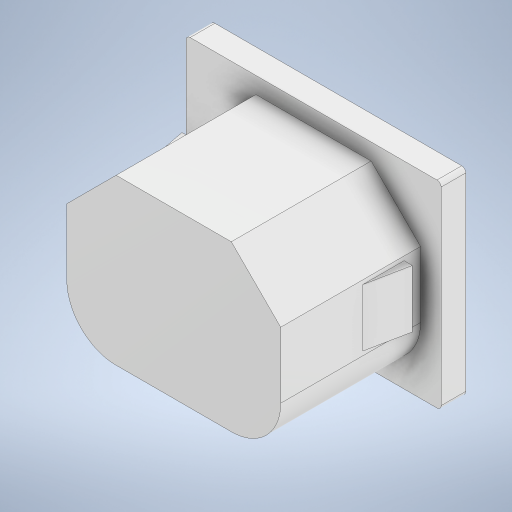
# Autodesk Inventor part: power_socket_24V_2
Saved by Autodesk Inventor 2023 (Build 270158000, 158)
## iProperties
Created: 2023-06-03
Part Number: power_socket_24V_2
Material: ABS Plastic
Document SubType Name: Modeling
Designer: 310611102
Density: 1.06 g/cm^3
Appearance: Smooth - White
Mass: 3.9038 g
Surface Area: 48.2017 cm^2
Volume: 3.68283 cm^3
Author: 310611102
Autodesk Inventor part; units mm, degrees
ref_plane "YZ Plane" through (0, 0, 0) normal (1, 0, 0) x (0, 1, 0)
ref_plane "XZ Plane" through (0, 0, 0) normal (0, 1, 0) x (-1, 0, 0)
ref_plane "XY Plane" through (0, 0, 0) normal (0, 0, 1) x (1, 0, 0)
sketch "Sketch1" plane through (0, 0, 0) normal (0, 0, 1) x (1, 0, 0)
  line L0 (-15.5, 12) -> (15.5, 12)
  line L1 (15.5, 12) -> (15.5, -12)
  line L2 (15.5, -12) -> (-15.5, -12)
  line L3 (-15.5, -12) -> (-15.5, 12)
  line L4 (-15.5, 12) -> (15.5, -12) construction
  line L5 (15.5, 12) -> (-15.5, -12) construction
  point P0 (0, 0)
  dimension "d0" = 24
  dimension "d1" = 31
  constraints: 12 end point, 8 point on line, 2 midpoint, 2 parallel, 1 horizontal, 1 perpendicular
  measures "d0" distance of L5.start L4.end
  measures "d1" distance of L4.start L5.start
extrude "Extrusion1" add sketch "Sketch1" along normal blind 3
fillet "Fillet1" radius 0.5 4 edges at (15.5, 12, 1.5) (15.5, -12, 1.5) (-15.5, -12, 1.5) (-15.5, 12, 1.5)
sketch "Sketch4" plane through (0, 0, 3) normal (0, 0, 1) x (1, 0, 0)
  line L0 (-7, -10) -> (7, -10)
  line L1 (13, -4) -> (13, 4)
  line L2 (7, 10) -> (-7, 10)
  line L3 (-13, 4) -> (-13, -4)
  line L4 (-13, -10) -> (13, 10) construction
  line L5 (13, -10) -> (-13, 10) construction
  arc A0 (-13, -4) -> (-7, -10) centre (-7, -4) ccw
  arc A1 (7, -10) -> (13, -4) centre (7, -4) ccw
  line L6 (-7, 10) -> (-13, 4)
  line L7 (13, 4) -> (7, 10)
  point P0 (0, 0)
  point P1 (0, 0)
  dimension "d13" = 20
  dimension "d14" = 26
  dimension "d41" = 6
  dimension "d42" = 6
  dimension "d43" = 6
  dimension "d44" = 6
  dimension "d45" = 6
  constraints: 16 end point, 16 point on line, 4 point on circle, 4 tangent, 2 centre point, 2 midpoint, 2 parallel, 1 coincident, 1 equal radius, 1 horizontal, 1 perpendicular
  measures "d13" distance of L5.start L4.end
  measures "d14" distance of L4.end L5.end
  measures "d41" radius of A0
  measures "d42" distance of L2.end point (-13, 10)
  measures "d43" distance of L3.start point (-13, 10)
  measures "d44" distance of L1.end point (13, 10)
  measures "d45" distance of L2.start point (13, 10)
extrude "Extrusion4" add sketch "Sketch4" along normal blind 17
sketch "Sketch8" plane through (0, 0, 0) normal (0, 1, 0) x (-1, 0, 0)
  line L0 (-13, 10) -> (-14, 5)
  line L1 (-14, 5) -> (-13, 5)
  line L2 (-15, 3) -> (15, 3) projected
  line L3 (-13, 5) -> (-13, 10)
  line L4 (-13, 3) -> (-13, 20) projected
  point P0 (0, 0)
  dimension "d36" = 2
  dimension "d37" = 1
  dimension "d38" = 5
  constraints: 6 end point, 1 horizontal, 1 point on line, 1 vertical
  measures "d36" distance between parallel lines of L2 L1
  measures "d37" distance of L0.end L1.end
  measures "d38" distance of L1.end L0.start
extrude "Extrusion7" add sketch "Sketch8" along normal mid plane 7
mirror "Mirror1" about plane through (0, 0, 0) normal (1, 0, 0) of "Extrusion7"
sketch "Sketch5" plane through (0, 0, 0) normal (0, 0, -1) x (-1, 0, 0)
  line L0 (-7.5, 8.5) -> (7.5, 8.5)
  line L1 (12.5, 3.5) -> (12.5, -4.5)
  line L2 (8.5, -8.5) -> (-8.5, -8.5)
  line L3 (-12.5, -4.5) -> (-12.5, 3.5)
  line L4 (-12.5, 8.5) -> (12.5, -8.5) construction
  line L5 (12.5, 8.5) -> (-12.5, -8.5) construction
  line L6 (-12.5, 3.5) -> (-7.5, 8.5)
  line L7 (7.5, 8.5) -> (12.5, 3.5)
  arc A0 (-12.5, -4.5) -> (-8.5, -8.5) centre (-8.5, -4.5) ccw
  arc A1 (8.5, -8.5) -> (12.5, -4.5) centre (8.5, -4.5) ccw
  point P0 (0, 0)
  dimension "d18" = 17
  dimension "d19" = 25
  dimension "d20" = 5
  dimension "d21" = 5
  dimension "d22" = 5
  dimension "d23" = 5
  dimension "d24" = 4
  constraints: 16 end point, 8 point on line, 4 point on circle, 4 tangent, 2 centre point, 2 midpoint, 2 parallel, 1 equal radius, 1 horizontal, 1 perpendicular
  measures "d18" distance of L5.start L4.end
  measures "d19" distance of L4.start L5.start
  measures "d20" distance of L3.end L4.start
  measures "d21" distance of L0.start L4.start
  measures "d22" distance of L0.end L5.start
  measures "d23" distance of L1.start L5.start
  measures "d24" radius of A0
extrude "Extrusion5" cut sketch "Sketch5" against normal blind 17
sketch "Sketch7" plane through (0, 0, 17) normal (0, 0, -1) x (-1, 0, 0)
  line L0 (0.5, 3.7551) -> (-0.5, 3.7551)
  line L1 (-0.5, 3.7551) -> (-0.5, 0.5551)
  line L2 (-0.5, 0.5551) -> (0.5, 0.5551)
  line L3 (0.5, 0.5551) -> (0.5, 3.7551)
  line L4 (0.5, 3.7551) -> (-0.5, 0.5551) construction
  line L5 (-0.5, 3.7551) -> (0.5, 0.5551) construction
  line L6 (7.6155, -0.4449) -> (6.6155, -0.4449)
  line L7 (6.6155, -0.4449) -> (6.6155, -3.6449)
  line L8 (6.6155, -3.6449) -> (7.6155, -3.6449)
  line L9 (7.6155, -3.6449) -> (7.6155, -0.4449)
  line L10 (7.6155, -0.4449) -> (6.6155, -3.6449) construction
  line L11 (6.6155, -0.4449) -> (7.6155, -3.6449) construction
  line L12 (0, 0) -> (0, -2.165)
  line L13 (-7.6155, -0.4449) -> (-6.6155, -0.4449)
  line L14 (-6.6155, -0.4449) -> (-6.6155, -3.6449)
  line L15 (-6.6155, -3.6449) -> (-7.6155, -3.6449)
  line L16 (-7.6155, -3.6449) -> (-7.6155, -0.4449)
  line L17 (-7.6155, -0.4449) -> (-6.6155, -3.6449) construction
  line L18 (-6.6155, -0.4449) -> (-7.6155, -3.6449) construction
  point P0 (0, 2.1551)
  point P1 (7.1155, -2.0449)
  point P2 (-7.1155, -2.0449)
  point P3 (-7.1155, -0.4449)
  dimension "d27" = 1
  dimension "d28" = 1
  dimension "d29" = 3.2
  dimension "d30" = 3.2
  dimension "d35" = 1
  constraints: 38 end point, 5 midpoint, 5 symmetric about line, 4 parallel, 2 horizontal, 2 perpendicular, 1 coincident, 1 vertical
  measures "d27" distance of L0.start L0.end
  measures "d28" distance of L13.start L13.end
  measures "d29" distance of L13.end L14.end
  measures "d30" distance of L2.end L0.start
  measures "d35" distance between parallel lines of L2 L13
extrude "Extrusion6" add sketch "Sketch7" along normal blind 14
equation "\"d43\" = d42"
equation "\"d44\" = d42"
equation "\"d45\" = d44"
equation "\"d21\" = d20"
equation "\"d22\" = d20"
equation "\"d23\" = d22"
body "Solid1"
